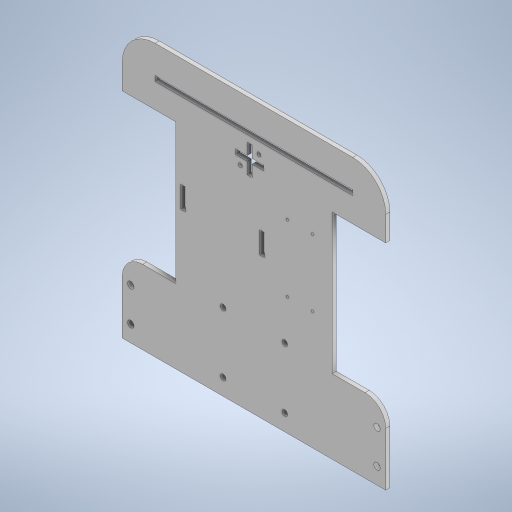
# Autodesk Inventor part: Peça1
Saved by Autodesk Inventor 2024.2 (Build 282272000, 272)
## iProperties
Created: 2024-04-09
Part Number: Peça1
Material: Genérico
Document SubType Name: Modeling
Designer: Documentos
Density: 1 g/cm^3
Appearance: Padrão
Author: Documentos
Autodesk Inventor part; units mm, degrees
ref_plane "YZ Plane" through (0, 0, 0) normal (1, 0, 0) x (0, 1, 0)
ref_plane "XZ Plane" through (0, 0, 0) normal (0, 1, 0) x (-1, 0, 0)
ref_plane "XY Plane" through (0, 0, 0) normal (0, 0, 1) x (1, 0, 0)
sketch "Esboço1" plane through (0, 0, 0) normal (0, 0, 1) x (1, 0, 0)
  line L0 (0, 0) -> (160, 0)
  line L1 (160, 0) -> (160, 32.5)
  line L2 (0, 32.5) -> (0, 0)
  line L3 (20, 165) -> (140, 165)
  line L4 (160, 145) -> (160, 130)
  line L5 (0, 130) -> (0, 145)
  arc A0 (20, 165) -> (0, 145) centre (20, 145) ccw
  arc A1 (160, 145) -> (140, 165) centre (140, 145) ccw
  line L6 (127.5, 130) -> (127.5, 45)
  line L7 (32.5, 45) -> (32.5, 130)
  line L8 (12.5, 45) -> (32.5, 45)
  line L9 (127.5, 45) -> (147.5, 45)
  line L10 (160, 130) -> (127.5, 130)
  line L11 (32.5, 130) -> (0, 130)
  arc A2 (12.5, 45) -> (0, 32.5) centre (12.5, 32.5) ccw
  arc A3 (160, 32.5) -> (147.5, 45) centre (147.5, 32.5) ccw
  line L12 (20, 148) -> (20, 145)
  line L13 (20, 145) -> (140, 145)
  line L14 (140, 145) -> (140, 148)
  line L15 (140, 148) -> (20, 148)
  point P0 (0, 165)
  point P1 (160, 165)
  dimension "d3" = 160
  dimension "d4" = 165
  dimension "d6" = 20
  dimension "d12" = 95
  dimension "d14" = 85
  dimension "d15" = 35
  dimension "d16" = 12.5
  dimension "d17" = 12.5
  dimension "d73" = 3
  dimension "d74" = 32.5
  constraints: 32 end point, 8 point on circle, 8 tangent, 7 perpendicular, 5 parallel, 4 centre point, 4 collinear, 4 point on line, 2 horizontal, 1 equal radius, 1 vertical
  measures "d3" distance of point (0, 165) point (160, 165)
  measures "d4" distance between parallel lines of L0 L3
  measures "d6" radius of A0
  measures "d12" distance between parallel lines of L6 L7
  measures "d14" distance between parallel lines of L9 L10
  measures "d15" distance between parallel lines of L3 L10
  measures "d16" radius of A2
  measures "d17" radius of A3
  measures "d73" distance between parallel lines of L13 L15
  measures "d74" distance between parallel lines of L5 L7
extrude "Extrusão1" add sketch "Esboço1" along normal blind 2.5
sketch "Esboço2" plane through (0, 0, 0) normal (0, 0, -1) x (-1, 0, 0)
  line L0 (-10.5, 30.486) -> (-10.5, 10)
  line L1 (-10.5, 10) -> (0, 10)
  line L2 (0, 10) -> (0, 30.486)
  line L3 (0, 30.486) -> (-10.5, 30.486)
  line L4 (0, 32.5) -> (0, 0) projected
  line L5 (0, 0) -> (-160, 0) projected
  line L6 (-160, 30.486) -> (-160, 10)
  line L7 (-160, 10) -> (-149.5, 10)
  line L8 (-149.5, 10) -> (-149.5, 30.486)
  line L9 (-149.5, 30.486) -> (-160, 30.486)
  line L10 (-160, 0) -> (-160, 32.5) projected
  circle A0 centre (-5.25, 10) radius 2
  circle A1 centre (-154.75, 30.486) radius 2
  circle A2 centre (-154.75, 10) radius 2
  circle A3 centre (-5.25, 30.486) radius 2
  line L11 (-98.69, 46.742) -> (-98.69, 10)
  line L12 (-98.69, 10) -> (-61.31, 10)
  line L13 (-61.31, 10) -> (-61.31, 46.742)
  line L14 (-61.31, 46.742) -> (-98.69, 46.742)
  circle A4 centre (-98.69, 46.742) radius 1.75
  circle A5 centre (-61.31, 46.742) radius 1.75
  circle A6 centre (-98.69, 10) radius 1.75
  circle A7 centre (-61.31, 10) radius 1.75
  line L15 (-100.26, 112.382) -> (-115.5, 112.382)
  line L16 (-115.5, 112.382) -> (-115.5, 71.742)
  line L17 (-115.5, 71.742) -> (-100.26, 71.742)
  line L18 (-100.26, 71.742) -> (-100.26, 112.382)
  line L19 (-127.5, 45) -> (-127.5, 130) projected
  circle A8 centre (-100.26, 112.382) radius 0.75
  circle A9 centre (-115.5, 112.382) radius 0.75
  circle A10 centre (-115.5, 71.742) radius 0.75
  circle A11 centre (-100.26, 71.742) radius 0.75
  line L20 (-68.8516, 140.982) -> (-85.9516, 140.982)
  line L21 (-85.9516, 140.982) -> (-85.9516, 123.882)
  line L22 (-85.9516, 123.882) -> (-68.8516, 123.882)
  line L23 (-68.8516, 123.882) -> (-68.8516, 140.982)
  circle A12 centre (-83.0586, 138.0895) radius 1.25
  circle A13 centre (-71.7446, 126.775) radius 1.25
  line L24 (-32.5, 130) -> (-32.5, 45) projected
  line L25 (-83.5, 75.089) -> (-38.5, 75.089)
  line L26 (-38.5, 75.089) -> (-38.5, 109.089)
  line L27 (-38.5, 109.089) -> (-83.5, 109.089)
  line L28 (-83.5, 109.089) -> (-83.5, 75.089)
  line L29 (-38.5, 98.658) -> (-35.5, 98.658)
  line L30 (-35.5, 98.658) -> (-35.5, 85.52)
  line L31 (-35.5, 85.52) -> (-38.5, 85.52)
  line L32 (-83.5, 98.658) -> (-86.5, 98.658)
  line L33 (-86.5, 98.658) -> (-86.5, 85.52)
  line L34 (-86.5, 85.52) -> (-83.5, 85.52)
  line L35 (-68.8516, 133.932) -> (-75.9016, 133.932)
  line L36 (-78.9016, 133.932) -> (-85.9516, 133.932)
  line L37 (-85.9516, 130.932) -> (-78.9016, 130.932)
  line L38 (-75.9016, 130.932) -> (-68.8516, 130.932)
  line L39 (-75.9016, 140.982) -> (-75.9016, 133.932)
  line L40 (-75.9016, 130.932) -> (-75.9016, 123.882)
  line L41 (-78.9016, 123.882) -> (-78.9016, 130.932)
  line L42 (-78.9016, 133.932) -> (-78.9016, 140.982)
  dimension "d20" = 20.486
  dimension "d21" = 10.5
  dimension "d22" = 10
  dimension "d23" = 20.486
  dimension "d24" = 10.5
  dimension "d26" = 4
  dimension "d27" = 4
  dimension "d28" = 4
  dimension "d29" = 4
  dimension "d30" = 36.742
  dimension "d35" = 3.5
  dimension "d36" = 3.5
  dimension "d37" = 3.5
  dimension "d38" = 3.5
  dimension "d39" = 15.24
  dimension "d40" = 40.64
  dimension "d42" = 12
  dimension "d43" = 1.5
  dimension "d44" = 1.5
  dimension "d45" = 1.5
  dimension "d46" = 1.5
  dimension "d47" = 17.1
  dimension "d48" = 17.1
  dimension "d50" = 2.5
  dimension "d51" = 2.5
  dimension "d52" = 2.893
  dimension "d53" = 2.8925
  dimension "d54" = 2.893
  dimension "d55" = 2.893
  dimension "d56" = 36.3516
  dimension "d57" = 41.5484
  dimension "d58" = 11.5
  dimension "d59" = 45
  dimension "d60" = 34
  dimension "d64" = 6
  dimension "d65" = 3
  dimension "d66" = 10.431
  dimension "d67" = 10.431
  dimension "d68" = 3
  dimension "d79" = 3
  dimension "d80" = 3
  dimension "d81" = 7.05
  dimension "d82" = 7.05
  dimension "d83" = 28.347
  dimension "d84" = 25
  dimension "d85" = 10
  dimension "d86" = 50.81
  dimension "d87" = 50.81
  dimension "d88" = 37.38
  constraints: 76 end point, 18 perpendicular, 14 centre point, 12 parallel, 12 point on line, 9 collinear, 8 coincident, 4 horizontal, 4 midpoint
  measures "d20" distance of L2.end L1.end
  measures "d21" distance of L1.end L0.end
  measures "d22" distance between parallel lines of L5 L1
  measures "d23" distance of L8.end L7.end
  measures "d24" distance of L7.end L6.end
  measures "d26" diameter of A0
  measures "d27" diameter of A1
  measures "d28" diameter of A2
  measures "d29" diameter of A3
  measures "d30" distance of L13.end L12.end
  measures "d35" diameter of A4
  measures "d36" diameter of A5
  measures "d37" diameter of A6
  measures "d38" diameter of A7
  measures "d39" distance of L17.end L16.end
  measures "d40" distance of L16.end L15.end
  measures "d42" distance between parallel lines of L19 L16
  measures "d43" diameter of A8
  measures "d44" diameter of A9
  measures "d45" diameter of A10
  measures "d46" diameter of A11
  measures "d47" distance of L22.end L21.end
  measures "d48" distance of L21.end L20.end
  measures "d50" diameter of A12
  measures "d51" diameter of A13
  measures "d52" distance from line of L21 A12.centre
  measures "d53" distance from line of L20 A12.centre
  measures "d54" distance from line of L22 A13.centre
  measures "d55" distance from line of L23 A13.centre
  measures "d56" distance between parallel lines of L23 L24
  measures "d57" distance between parallel lines of L21 L19
  measures "d58" distance between parallel lines of L15 L22
  measures "d59" distance of L27.end L26.end
  measures "d60" distance between parallel lines of L27 L25
  measures "d64" distance between parallel lines of L26 L24
  measures "d65" distance of L29.start L29.end
  measures "d66" distance between parallel lines of L25 L31
  measures "d67" distance between parallel lines of L29 L27
  measures "d68" distance of L32.start L32.end
  measures "d79" distance between parallel lines of L38 L35
  measures "d80" distance between parallel lines of L41 L40
  measures "d81" distance between parallel lines of L21 L41
  measures "d82" distance between parallel lines of L22 L37
  measures "d83" distance between parallel lines of L14 L25
  measures "d84" distance between parallel lines of L14 L17
  measures "d85" distance between parallel lines of L5 L12
  measures "d86" distance between parallel lines of L0 L13
  measures "d87" distance between parallel lines of L8 L11
  measures "d88" distance of L12.end L11.end
extrude "Extrusão2" cut sketch "Esboço2" against normal through all contours A3 L3 | L3 A3 | A0 L1 | L1 A0 | A2 L7 | L7 A2 | A1 L9 | L9 A1 | L14 A4 L11 | L11 A4 L14 | A6 L12 L11 | L11 L12 A6 | A5 L13 L14 | L14 L13 A5 | A7 L13 L12 | L12 L13 A7 | A9 L16 L15 | L15 L16 A9 | A8 L18 L15 | L15 L18 A8 | A10 L17 L16 | L16 L17 A10 | A11 L17 L18 | L18 L17 A11 | L39 L35 L23 L38 L40 L22 L41 L37 L21 L36 L42 L20 | A12 | A13 | L34 L33 L32 L28 | L26 L29 L30 L31
